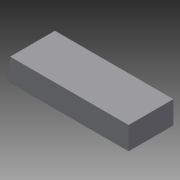
# Autodesk Inventor part: FelixOriginalBearingHolder
Saved by Autodesk Inventor 2015 SP1 (Build 190203100, 203)
## iProperties
Created: 2014-12-14
Part Number: FelixOriginalBearingHolder
Material: Generic
Document SubType Name: Modeling
Designer: Jack
Density: 1 g/cm^3
Appearance: Default
Author: Jack
Autodesk Inventor part; units mm, degrees
ref_plane "YZ Plane" through (0, 0, 0) normal (1, 0, 0) x (0, 1, 0)
ref_plane "XZ Plane" through (0, 0, 0) normal (0, 1, 0) x (-1, 0, 0)
ref_plane "XY Plane" through (0, 0, 0) normal (0, 0, 1) x (1, 0, 0)
sketch "Sketch1" plane through (0, 0, 0) normal (0, 0, 1) x (1, 0, 0)
  line L0 (0, 0) -> (36.8834, 238.252)
  line L1 (36.8834, 238.252) -> (1278.89, 238.252)
  line L2 (1278.89, 238.252) -> (1278.89, 0)
  line L3 (1278.89, 0) -> (0, 0)
  dimension "d2" = 1278.89
  dimension "d3" = 81.2
  dimension "d4" = 238.252
  constraints: 8 end point, 2 perpendicular, 1 horizontal
  measures "d2" distance of L2.end L0.start
  measures "d3" angle of L3 L0
  measures "d4" distance of L1.end L2.end
extrude "Extrusion1" add sketch "Sketch1" along normal blind 469.9
body "Solid1"
